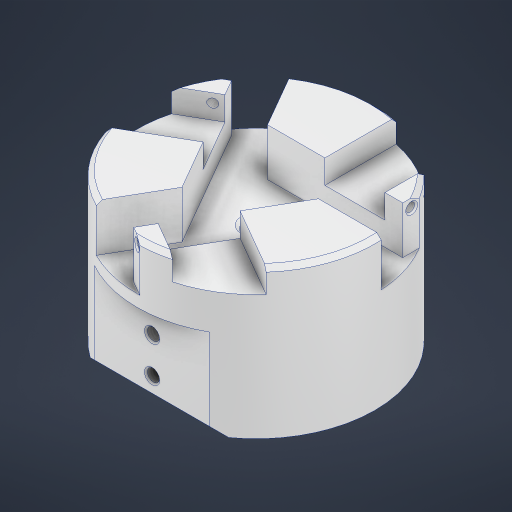
# Autodesk Inventor part: BaseSupport
Saved by Autodesk Inventor 2023 (Build 270158000, 158)
## iProperties
Created: 2023-02-24
Part Number: BaseSupport
Material: Aluminum 6061
Document SubType Name: Modeling
Designer: roota
Density: 2.7 g/cm^3
Appearance: Aluminum - Flat
Mass: 612.501 g
Surface Area: 232.858 cm^2
Volume: 226.852 cm^3
Author: roota
Autodesk Inventor part; units mm, degrees
ref_plane "YZ Plane" through (0, 0, 0) normal (1, 0, 0) x (0, 1, 0)
ref_plane "XZ Plane" through (0, 0, 0) normal (0, 1, 0) x (-1, 0, 0)
ref_plane "XY Plane" through (0, 0, 0) normal (0, 0, 1) x (1, 0, 0)
sketch "Sketch1" plane through (0, 0, 0) normal (0, 1, 0) x (-1, 0, 0)
  circle A0 centre (0, 0) radius 70 construction
  line L0 (32.2622, 28.3815) -> (0.4069, 28.3815) construction
  line L1 (0.4069, 28.3815) -> (0.4069, 1.4276) construction
  line L2 (0.4069, 1.4276) -> (32.2622, 1.4276) construction
  line L3 (32.2622, 1.4276) -> (32.2622, 28.3815) construction
  line L4 (21.4142, 1.4276) -> (78.1619, 1.4276) construction
  line L5 (78.1619, 1.4276) -> (78.1619, -1.5168) construction
  line L6 (78.1619, -1.5168) -> (21.4142, -1.5168) construction
  line L7 (21.4142, -1.5168) -> (21.4142, 1.4276) construction
  line L8 (8.448, -42.1306) -> (24.3757, -14.5431) construction
  line L9 (24.3757, -14.5431) -> (1.0329, -1.0662) construction
  line L10 (1.0329, -1.0662) -> (-14.8947, -28.6537) construction
  line L11 (-14.8947, -28.6537) -> (8.448, -42.1306) construction
  line L12 (-9.4708, -19.2591) -> (-37.8446, -68.404) construction
  line L13 (-37.8446, -68.404) -> (-40.3946, -66.9318) construction
  line L14 (-40.3946, -66.9318) -> (-12.0207, -17.7868) construction
  line L15 (-12.0207, -17.7868) -> (-9.4708, -19.2591) construction
  line L16 (-40.7102, 13.7491) -> (-24.7826, -13.8384) construction
  line L17 (-24.7826, -13.8384) -> (-1.4398, -0.3614) construction
  line L18 (-1.4398, -0.3614) -> (-17.3674, 27.2261) construction
  line L19 (-17.3674, 27.2261) -> (-40.7102, 13.7491) construction
  line L20 (-11.9435, 17.8314) -> (-40.3173, 66.9764) construction
  line L21 (-40.3173, 66.9764) -> (-37.7673, 68.4486) construction
  line L22 (-37.7673, 68.4486) -> (-9.3935, 19.3037) construction
  line L23 (-9.3935, 19.3037) -> (-11.9435, 17.8314) construction
  circle A1 centre (0, 0) radius 40
  dimension "d0" = 140
  dimension "d3" = 360
  dimension "d5" = 80
  constraints: 48 end point, 6 coincident, 4 parallel, 3 point on line, 2 centre point, 2 horizontal, 2 perpendicular, 53 other
  measures "d0" diameter of A0
  measures "d5" diameter of A1
extrude "Extrusion1" add sketch "Sketch1" along normal blind 50
sketch "Sketch2" plane through (0, 50, 0) normal (0, 1, 0) x (1, 0, 0)
  circle A0 centre (0, 0) radius 40 projected
  line L0 (-19.3649, -35) -> (19.3649, -35)
  line L1 (-19.3649, 35) -> (19.3649, 35)
  point P0 (0, -35)
  dimension "d8" = 70
  constraints: 4 end point, 4 point on circle, 2 parallel, 1 horizontal, 1 midpoint
  measures "d8" distance from line of point (0, -35) L1
extrude "Extrusion2" cut sketch "Sketch2" along normal blind 30 from surface at -50 contours L1 A0 | A0 L0
sketch "Sketch3" plane through (-19.3649, 50, 35) normal (0, 0, 1) x (1, 0, 0)
  line L0 (38.7298, -50) -> (0, -50) projected
  point P0 (19.3649, -50)
  point P1 (19.3649, -42.5)
  point P2 (19.3649, -50)
  point P3 (19.3649, -30.5)
  point P4 (19.3649, -50)
  dimension "d11" = 7.5
  dimension "d12" = 12
  constraints: 2 midpoint, 2 vertical alignment
  measures "d11" distance of point (19.365, -50) point (19.365, -42.5)
  measures "d12" distance of point (19.365, -42.5) point (19.365, -30.5)
hole "Hole1" at (0, 7.5, 35) at (0, 19.5, 35) direction (0, 0, -1) diameter 4.134 depth 15 tip angle 118 thread size "M5x0.8" class "6H" standard "ISO Metric profile"
mirror "Mirror1" about plane through (0, 0, 0) normal (0, 0, 1) of "Hole1"
chamfer "Chamfer1" distance 2.5 angle 45 2 edges at (0, 0, 35) (0, 0, -35)
sketch "Sketch4" plane through (0, 50, 0) normal (0, 1, 0) x (1, 0, 0)
  line L0 (8, 2.2) -> (52.7697, 2.2)
  line L1 (52.7697, 2.2) -> (52.7697, 51.6778)
  line L2 (52.7697, 51.6778) -> (8, 51.6778)
  line L3 (8, 51.6778) -> (8, 2.2)
  line L4 (19.3649, 35) -> (-19.3649, 35) projected
  point P0 (0, 0)
  dimension "d25" = 8
  dimension "d26" = 32.8
  constraints: 8 end point, 2 parallel, 1 horizontal, 1 perpendicular
  measures "d25" distance from line of point (0, 0) L3
  measures "d26" distance between parallel lines of L4 L0
extrude "Extrusion3" cut sketch "Sketch4" against normal blind 8
sketch "Sketch5" plane through (0, 50, 0) normal (0, 1, 0) x (1, 0, 0)
  circle A0 centre (0, 0) radius 15.2
  dimension "d30" = 30.4
  constraints: 1 centre point, 1 coincident
  measures "d30" diameter of A0
extrude "Extrusion4" cut sketch "Sketch5" against normal blind 16
sketch "Sketch6" plane through (0, 42, 0) normal (0, 1, 0) x (1, 0, 0)
  line L0 (0, 6.2) -> (49.6496, 6.2)
  line L1 (49.6496, 6.2) -> (49.6496, 15.2)
  line L2 (49.6496, 15.2) -> (0, 15.2)
  line L3 (0, 15.2) -> (0, 6.2)
  line L4 (39.9395, 2.2) -> (15.0399, 2.2) projected
  line L5 (8, 12.9244) -> (8, 39.1918) projected
  line L6 (0, 0) -> (15.2, 0)
  line L7 (15.2, 0) -> (15.2, 6.2)
  line L8 (15.2, 6.2) -> (0, 6.2)
  line L9 (0, 6.2) -> (0, 0)
  point P0 (0, 0)
  point P1 (8, 35)
  dimension "d33" = 9
  dimension "d34" = 4
  dimension "d39" = 15.2
  constraints: 16 end point, 4 parallel, 2 horizontal, 2 perpendicular, 1 coincident, 1 point on line, 1 vertical alignment
  measures "d33" distance of L0.end L1.end
  measures "d34" distance between parallel lines of L4 L0
  measures "d39" distance from line of point (0, 0) L7
extrude "Extrusion5" cut sketch "Sketch6" along normal blind 20.75 and the other way blind 8
pattern_circular "Circular Pattern2" count 3 over 360 about axis through (0, 0, 0) along (0, 1, 0) of "Extrusion3", "Extrusion5"
sketch "Sketch7" plane through (0, 50, 0) normal (0, 1, 0) x (1, 0, 0)
  line L0 (8, 15.2) -> (36.9995, 15.2) projected
  arc A0 (39.9395, 2.2) -> (39.5166, 6.2) centre (0, 0) ccw projected
  line L1 (8, 15.2) -> (8, 39.1918) projected
  arc A1 (-31.6633, 24.4425) -> (-37.9411, -12.6677) centre (0, 0) ccw projected
  line L2 (-17.1636, -0.6718) -> (-37.9411, -12.6677) projected
  line L3 (-31.6633, 24.4425) -> (-17.1636, -0.6718) projected
  arc A2 (-5.3361, -39.6425) -> (29.9411, -26.5241) centre (0, 0) ccw projected
  line L4 (9.1636, -14.5282) -> (29.9411, -26.5241) projected
  line L5 (-5.3361, -39.6425) -> (9.1636, -14.5282) projected
  line L6 (28.2, 28.3683) -> (28.2, 15.2)
  line L7 (0, 15.2) -> (36.9995, 15.2) projected
  line L8 (34.2, 15.2) -> (34.2, 20.7451)
  arc A3 (36.9995, 15.2) -> (8, 39.1918) centre (0, 0) ccw projected
  line L9 (15.2, 6.2) -> (15.2, 2.2) projected
  line L10 (39.9395, 2.2) -> (15.2, 2.2) projected
  line L11 (39.5166, 6.2) -> (15.2, 6.2) projected
  arc A4 (-18.0645, -35.6886) -> (-14.3889, -37.3224) centre (0, 0) ccw projected
  line L12 (-2.2306, -16.2636) -> (-14.3889, -37.3224) projected
  line L13 (-5.6947, -14.2636) -> (-2.2306, -16.2636) projected
  line L14 (-18.0645, -35.6886) -> (-5.6947, -14.2636) projected
  dimension "d43" = 20.2
  dimension "d46" = 6
  constraints: 4 end point, 2 perpendicular, 2 point on circle, 2 point on line
  measures "d43" distance between parallel lines of L1 L6
  measures "d46" distance between parallel lines of L6 L8
extrude "Extrusion6" add sketch "Sketch7" along normal blind 8 from surface at -8 contours L6 A3 L8 L0 | L10 L9 L11 A0
sketch "Sketch8" plane through (34.2, 50, -15.2) normal (1, 0, 0) x (0, 0, -1)
  circle A0 centre (3, -3) radius 1.5
  line L0 (0, -8) -> (0, 0) projected
  line L1 (0, 0) -> (5.5451, 0) projected
  point P0 (-15.2, -50)
  dimension "d47" = 3
  dimension "d48" = 3
  dimension "d51" = 3
  constraints: 1 centre point
  measures "d47" diameter of A0
  measures "d48" distance from line of L0 A0.centre
  measures "d51" distance from line of L1 A0.centre
extrude "Extrusion7" cut sketch "Sketch8" against normal blind 10
thread "Thread1" size "M3x0.5" class "6H" standard "ISO Metric profile" length 15
extrude "Extrusion8" cut sketch "Sketch7" against normal up to surface (16 mm away) contours L8 A3 L0 | L10 L9 L11 A0
pattern_circular "Circular Pattern3" count 3 over 360 about axis through (0, 0, 0) along (0, 1, 0) of "Extrusion6", "Extrusion7", "Extrusion8"
sketch "Sketch9" plane through (0, 50, 0) normal (0, 1, 0) x (1, 0, 0)
  line L0 (26.3272, 15.2) -> (-26.3272, 15.2)
  line L1 (-26.3272, 15.2) -> (0, -30.4)
  line L2 (0, -30.4) -> (26.3272, 15.2)
  line L3 (-0.9364, -32.0219) -> (9.1636, -14.5282) projected
  line L4 (-27.2636, 16.8219) -> (-17.1636, -0.6718) projected
  point P0 (0, 0)
  point P1 (0, 15.2)
  point P2 (-13.1636, -7.6)
  point P3 (13.1636, -7.6)
  constraints: 6 end point, 3 midpoint, 2 point on line, 1 horizontal
extrude "Extrusion9" cut sketch "Sketch9" against normal up to surface (16 mm away)
sketch "Sketch10" plane through (0, 34, 0) normal (0, 1, 0) x (1, 0, 0)
  circle A0 centre (0, 0) radius 4
  dimension "d61" = 8
  constraints: 1 centre point, 1 coincident
  measures "d61" diameter of A0
extrude "Extrusion10" cut sketch "Sketch10" against normal blind 41.25
thread "Thread2" size "M8x1.25" class "6H" standard "ANSI Metric M Profile" length 15
chamfer "Chamfer2" distance 1 angle 45 1 edges at (-4, 34, 0)
chamfer "Chamfer3" distance 0.5 angle 45 7 edges at (34.2, 47, -16.7) (-2.6374, 47, 37.9681) (-31.5626, 47, -21.2681) (0, 21.567, 35) (0, 9.567, 35) (0, 21.567, -35) (0, 9.567, -35)
chamfer "Chamfer4" distance 1.5 angle 45 6 edges at (37.7769, 50, 13.1494) (5.7089, 50, 39.5905) (-30.2762, 50, 26.141) (-37.1408, 50, -14.8512) (-7.5007, 50, -39.2904) (31.432, 50, -24.7393)
body "Solid1"
